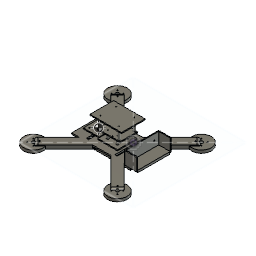
Drone Prototype Cad Model (Autodesk Fusion 360 design; units mm, degrees)
Autodesk Fusion 360 part; units mm, degrees
ref_plane "WorkPlane1" through (0, 0, 0) normal (0, 0, 1) x (1, 0, 0) in component "Standard_X_7in_Drone_OAKD_Pixhawk_Pi5_Final_Concept"
sketch "Arm_1_sketch" plane through (0, 0, 0) normal (0, 0, 1) x (1, 0, 0) in component "Standard_X_7in_Drone_OAKD_Pixhawk_Pi5_Final_Concept"
  line L0 (-10.6066, 10.6066) -> (121.9759, 143.1891)
  line L1 (121.9759, 143.1891) -> (143.1891, 121.9759)
  line L2 (143.1891, 121.9759) -> (10.6066, -10.6066)
  line L3 (10.6066, -10.6066) -> (-10.6066, 10.6066)
extrude "Extrude1" add sketch "Arm_1_sketch" along normal blind 12 makes body 1 in component "Standard_X_7in_Drone_OAKD_Pixhawk_Pi5_Final_Concept"
ref_plane "WorkPlane2" through (0, 0, 0) normal (0, 0, 1) x (1, 0, 0) in component "Standard_X_7in_Drone_OAKD_Pixhawk_Pi5_Final_Concept"
sketch "Arm_2_sketch" plane through (0, 0, 0) normal (0, 0, 1) x (1, 0, 0) in component "Standard_X_7in_Drone_OAKD_Pixhawk_Pi5_Final_Concept"
  line L0 (10.6066, 10.6066) -> (143.1891, -121.9759)
  line L1 (143.1891, -121.9759) -> (121.9759, -143.1891)
  line L2 (121.9759, -143.1891) -> (-10.6066, -10.6066)
  line L3 (-10.6066, -10.6066) -> (10.6066, 10.6066)
extrude "Extrude2" add sketch "Arm_2_sketch" along normal blind 12 separate body makes body 2 in component "Standard_X_7in_Drone_OAKD_Pixhawk_Pi5_Final_Concept"
ref_plane "WorkPlane3" through (0, 0, 0) normal (0, 0, 1) x (1, 0, 0) in component "Standard_X_7in_Drone_OAKD_Pixhawk_Pi5_Final_Concept"
sketch "Arm_3_sketch" plane through (0, 0, 0) normal (0, 0, 1) x (1, 0, 0) in component "Standard_X_7in_Drone_OAKD_Pixhawk_Pi5_Final_Concept"
  line L0 (10.6066, -10.6066) -> (-121.9759, -143.1891)
  line L1 (-121.9759, -143.1891) -> (-143.1891, -121.9759)
  line L2 (-143.1891, -121.9759) -> (-10.6066, 10.6066)
  line L3 (-10.6066, 10.6066) -> (10.6066, -10.6066)
extrude "Extrude3" add sketch "Arm_3_sketch" along normal blind 12 separate body makes body 3 in component "Standard_X_7in_Drone_OAKD_Pixhawk_Pi5_Final_Concept"
ref_plane "WorkPlane4" through (0, 0, 0) normal (0, 0, 1) x (1, 0, 0) in component "Standard_X_7in_Drone_OAKD_Pixhawk_Pi5_Final_Concept"
sketch "Arm_4_sketch" plane through (0, 0, 0) normal (0, 0, 1) x (1, 0, 0) in component "Standard_X_7in_Drone_OAKD_Pixhawk_Pi5_Final_Concept"
  line L0 (-10.6066, -10.6066) -> (-143.1891, 121.9759)
  line L1 (-143.1891, 121.9759) -> (-121.9759, 143.1891)
  line L2 (-121.9759, 143.1891) -> (10.6066, 10.6066)
  line L3 (10.6066, 10.6066) -> (-10.6066, -10.6066)
extrude "Extrude4" add sketch "Arm_4_sketch" along normal blind 12 separate body makes body 4 in component "Standard_X_7in_Drone_OAKD_Pixhawk_Pi5_Final_Concept"
ref_plane "WorkPlane5" through (0, 0, 0) normal (0, 0, 1) x (1, 0, 0) in component "Standard_X_7in_Drone_OAKD_Pixhawk_Pi5_Final_Concept"
sketch "Motor_Pad_1_sketch" plane through (0, 0, 0) normal (0, 0, 1) x (1, 0, 0) in component "Standard_X_7in_Drone_OAKD_Pixhawk_Pi5_Final_Concept"
  circle A0 centre (132.5825, 132.5825) radius 31
extrude "Extrude5" add sketch "Motor_Pad_1_sketch" along normal blind 9 separate body makes body 5 in component "Standard_X_7in_Drone_OAKD_Pixhawk_Pi5_Final_Concept"
ref_plane "WorkPlane6" through (0, 0, 0) normal (0, 0, 1) x (1, 0, 0) in component "Standard_X_7in_Drone_OAKD_Pixhawk_Pi5_Final_Concept"
sketch "Motor_Pad_2_sketch" plane through (0, 0, 0) normal (0, 0, 1) x (1, 0, 0) in component "Standard_X_7in_Drone_OAKD_Pixhawk_Pi5_Final_Concept"
  circle A0 centre (132.5825, -132.5825) radius 31
extrude "Extrude6" add sketch "Motor_Pad_2_sketch" along normal blind 9 separate body makes body 6 in component "Standard_X_7in_Drone_OAKD_Pixhawk_Pi5_Final_Concept"
ref_plane "WorkPlane7" through (0, 0, 0) normal (0, 0, 1) x (1, 0, 0) in component "Standard_X_7in_Drone_OAKD_Pixhawk_Pi5_Final_Concept"
sketch "Motor_Pad_3_sketch" plane through (0, 0, 0) normal (0, 0, 1) x (1, 0, 0) in component "Standard_X_7in_Drone_OAKD_Pixhawk_Pi5_Final_Concept"
  circle A0 centre (-132.5825, -132.5825) radius 31
extrude "Extrude7" add sketch "Motor_Pad_3_sketch" along normal blind 9 separate body makes body 7 in component "Standard_X_7in_Drone_OAKD_Pixhawk_Pi5_Final_Concept"
ref_plane "WorkPlane8" through (0, 0, 0) normal (0, 0, 1) x (1, 0, 0) in component "Standard_X_7in_Drone_OAKD_Pixhawk_Pi5_Final_Concept"
sketch "Motor_Pad_4_sketch" plane through (0, 0, 0) normal (0, 0, 1) x (1, 0, 0) in component "Standard_X_7in_Drone_OAKD_Pixhawk_Pi5_Final_Concept"
  circle A0 centre (-132.5825, 132.5825) radius 31
extrude "Extrude8" add sketch "Motor_Pad_4_sketch" along normal blind 9 separate body makes body 8 in component "Standard_X_7in_Drone_OAKD_Pixhawk_Pi5_Final_Concept"
ref_plane "WorkPlane9" through (0, 0, 8) normal (0, 0, 1) x (1, 0, 0) in component "Standard_X_7in_Drone_OAKD_Pixhawk_Pi5_Final_Concept"
sketch "Central_Lower_Body_Plate_sketch" plane through (0, 0, 8) normal (0, 0, 1) x (1, 0, 0) in component "Standard_X_7in_Drone_OAKD_Pixhawk_Pi5_Final_Concept"
  line L0 (-95, -50) -> (115, -50)
  line L1 (115, -50) -> (115, 50)
  line L2 (115, 50) -> (-95, 50)
  line L3 (-95, 50) -> (-95, -50)
  dimension "d213" = 95
  dimension "d214" = 50
  dimension "d215" = 210
  dimension "d216" = 100
  constraint perpendicular L0 L3
  constraint perpendicular L0 L1
  constraint perpendicular L1 L2
  constraint coincident L0.start L3.end
  constraint coincident L2.end L3.start
  constraint coincident L0.end L1.start
  constraint coincident L1.end L2.start
  constraint vertical L1
  measures "d213" distance of origin L3
  measures "d214" distance of origin L0
  measures "d215" distance of L1 L3
  measures "d216" distance of L0 L2
extrude "Extrude9" add sketch "Central_Lower_Body_Plate_sketch" along normal blind 4 separate body makes body 9 in component "Standard_X_7in_Drone_OAKD_Pixhawk_Pi5_Final_Concept"
ref_plane "WorkPlane10" through (0, 0, -18) normal (0, 0, 1) x (1, 0, 0) in component "Standard_X_7in_Drone_OAKD_Pixhawk_Pi5_Final_Concept"
sketch "Battery_Left_Rail_sketch" plane through (0, 0, -18) normal (0, 0, 1) x (1, 0, 0) in component "Standard_X_7in_Drone_OAKD_Pixhawk_Pi5_Final_Concept"
  line L0 (-83, -32) -> (67, -32)
  line L1 (67, -32) -> (67, -26)
  line L2 (67, -26) -> (-83, -26)
  line L3 (-83, -26) -> (-83, -32)
extrude "Extrude10" add sketch "Battery_Left_Rail_sketch" along normal blind 16 separate body makes body 10 in component "Standard_X_7in_Drone_OAKD_Pixhawk_Pi5_Final_Concept"
ref_plane "WorkPlane11" through (0, 0, -18) normal (0, 0, 1) x (1, 0, 0) in component "Standard_X_7in_Drone_OAKD_Pixhawk_Pi5_Final_Concept"
sketch "Battery_Right_Rail_sketch" plane through (0, 0, -18) normal (0, 0, 1) x (1, 0, 0) in component "Standard_X_7in_Drone_OAKD_Pixhawk_Pi5_Final_Concept"
  line L0 (-83, 26) -> (67, 26)
  line L1 (67, 26) -> (67, 32)
  line L2 (67, 32) -> (-83, 32)
  line L3 (-83, 32) -> (-83, 26)
extrude "Extrude11" add sketch "Battery_Right_Rail_sketch" along normal blind 16 separate body makes body 11 in component "Standard_X_7in_Drone_OAKD_Pixhawk_Pi5_Final_Concept"
ref_plane "WorkPlane12" through (0, 0, -18) normal (0, 0, 1) x (1, 0, 0) in component "Standard_X_7in_Drone_OAKD_Pixhawk_Pi5_Final_Concept"
sketch "Battery_Front_Stop_sketch" plane through (0, 0, -18) normal (0, 0, 1) x (1, 0, 0) in component "Standard_X_7in_Drone_OAKD_Pixhawk_Pi5_Final_Concept"
  line L0 (67, -32) -> (73, -32)
  line L1 (73, -32) -> (73, 32)
  line L2 (73, 32) -> (67, 32)
  line L3 (67, 32) -> (67, -32)
extrude "Extrude12" add sketch "Battery_Front_Stop_sketch" along normal blind 16 separate body makes body 12 in component "Standard_X_7in_Drone_OAKD_Pixhawk_Pi5_Final_Concept"
ref_plane "WorkPlane13" through (0, 0, -18) normal (0, 0, 1) x (1, 0, 0) in component "Standard_X_7in_Drone_OAKD_Pixhawk_Pi5_Final_Concept"
sketch "Battery_Rear_Stop_sketch" plane through (0, 0, -18) normal (0, 0, 1) x (1, 0, 0) in component "Standard_X_7in_Drone_OAKD_Pixhawk_Pi5_Final_Concept"
  line L0 (-89, -32) -> (-83, -32)
  line L1 (-83, -32) -> (-83, 32)
  line L2 (-83, 32) -> (-89, 32)
  line L3 (-89, 32) -> (-89, -32)
extrude "Extrude13" add sketch "Battery_Rear_Stop_sketch" along normal blind 16 separate body makes body 13 in component "Standard_X_7in_Drone_OAKD_Pixhawk_Pi5_Final_Concept"
ref_plane "WorkPlane14" through (0, 0, -58) normal (0, 0, 1) x (1, 0, 0) in component "Standard_X_7in_Drone_OAKD_Pixhawk_Pi5_Final_Concept"
sketch "Battery_Mockup_SOCOKIN_6S_4000mAh_Do_Not_Print_sketch" plane through (0, 0, -58) normal (0, 0, 1) x (1, 0, 0) in component "Standard_X_7in_Drone_OAKD_Pixhawk_Pi5_Final_Concept"
  line L0 (-78, -21.5) -> (62, -21.5)
  line L1 (62, -21.5) -> (62, 21.5)
  line L2 (62, 21.5) -> (-78, 21.5)
  line L3 (-78, 21.5) -> (-78, -21.5)
extrude "Extrude14" add sketch "Battery_Mockup_SOCOKIN_6S_4000mAh_Do_Not_Print_sketch" along normal blind 49 separate body makes body 14 in component "Standard_X_7in_Drone_OAKD_Pixhawk_Pi5_Final_Concept"
ref_plane "WorkPlane15" through (0, 0, 16) normal (0, 0, 1) x (1, 0, 0) in component "Standard_X_7in_Drone_OAKD_Pixhawk_Pi5_Final_Concept"
sketch "Tekko32_ESC_Lower_Mounting_Deck_sketch" plane through (0, 0, 16) normal (0, 0, 1) x (1, 0, 0) in component "Standard_X_7in_Drone_OAKD_Pixhawk_Pi5_Final_Concept"
  line L0 (-31, -31) -> (31, -31)
  line L1 (31, -31) -> (31, 31)
  line L2 (31, 31) -> (-31, 31)
  line L3 (-31, 31) -> (-31, -31)
extrude "Extrude15" add sketch "Tekko32_ESC_Lower_Mounting_Deck_sketch" along normal blind 3 separate body makes body 15 in component "Standard_X_7in_Drone_OAKD_Pixhawk_Pi5_Final_Concept"
ref_plane "WorkPlane16" through (0, 0, 19) normal (0, 0, 1) x (1, 0, 0) in component "Standard_X_7in_Drone_OAKD_Pixhawk_Pi5_Final_Concept"
sketch "Tekko32_ESC_Mockup_Do_Not_Print_sketch" plane through (0, 0, 19) normal (0, 0, 1) x (1, 0, 0) in component "Standard_X_7in_Drone_OAKD_Pixhawk_Pi5_Final_Concept"
  line L0 (-25, -25) -> (25, -25)
  line L1 (25, -25) -> (25, 25)
  line L2 (25, 25) -> (-25, 25)
  line L3 (-25, 25) -> (-25, -25)
extrude "Extrude16" add sketch "Tekko32_ESC_Mockup_Do_Not_Print_sketch" along normal blind 12 separate body makes body 16 in component "Standard_X_7in_Drone_OAKD_Pixhawk_Pi5_Final_Concept"
ref_plane "WorkPlane17" through (0, 0, 16) normal (0, 0, 1) x (1, 0, 0) in component "Standard_X_7in_Drone_OAKD_Pixhawk_Pi5_Final_Concept"
sketch "PM06_Power_Module_Mounting_Deck_sketch" plane through (0, 0, 16) normal (0, 0, 1) x (1, 0, 0) in component "Standard_X_7in_Drone_OAKD_Pixhawk_Pi5_Final_Concept"
  line L0 (-83, -25) -> (-33, -25)
  line L1 (-33, -25) -> (-33, 25)
  line L2 (-33, 25) -> (-83, 25)
  line L3 (-83, 25) -> (-83, -25)
extrude "Extrude17" add sketch "PM06_Power_Module_Mounting_Deck_sketch" along normal blind 3 separate body makes body 17 in component "Standard_X_7in_Drone_OAKD_Pixhawk_Pi5_Final_Concept"
ref_plane "WorkPlane18" through (0, 0, 19) normal (0, 0, 1) x (1, 0, 0) in component "Standard_X_7in_Drone_OAKD_Pixhawk_Pi5_Final_Concept"
sketch "PM06_Power_Module_Mockup_Do_Not_Print_sketch" plane through (0, 0, 19) normal (0, 0, 1) x (1, 0, 0) in component "Standard_X_7in_Drone_OAKD_Pixhawk_Pi5_Final_Concept"
  line L0 (-79, -21) -> (-37, -21)
  line L1 (-37, -21) -> (-37, 21)
  line L2 (-37, 21) -> (-79, 21)
  line L3 (-79, 21) -> (-79, -21)
extrude "Extrude18" add sketch "PM06_Power_Module_Mockup_Do_Not_Print_sketch" along normal blind 12 separate body makes body 18 in component "Standard_X_7in_Drone_OAKD_Pixhawk_Pi5_Final_Concept"
ref_plane "WorkPlane19" through (0, 0, 12) normal (0, 0, 1) x (1, 0, 0) in component "Standard_X_7in_Drone_OAKD_Pixhawk_Pi5_Final_Concept"
sketch "ESC_Deck_Standoff_1_sketch" plane through (0, 0, 12) normal (0, 0, 1) x (1, 0, 0) in component "Standard_X_7in_Drone_OAKD_Pixhawk_Pi5_Final_Concept"
  circle A0 centre (-15.25, -15.25) radius 3.5
extrude "Extrude19" add sketch "ESC_Deck_Standoff_1_sketch" along normal blind 4 separate body makes body 19 in component "Standard_X_7in_Drone_OAKD_Pixhawk_Pi5_Final_Concept"
ref_plane "WorkPlane20" through (0, 0, 12) normal (0, 0, 1) x (1, 0, 0) in component "Standard_X_7in_Drone_OAKD_Pixhawk_Pi5_Final_Concept"
sketch "ESC_Deck_Standoff_2_sketch" plane through (0, 0, 12) normal (0, 0, 1) x (1, 0, 0) in component "Standard_X_7in_Drone_OAKD_Pixhawk_Pi5_Final_Concept"
  circle A0 centre (15.25, -15.25) radius 3.5
extrude "Extrude20" add sketch "ESC_Deck_Standoff_2_sketch" along normal blind 4 separate body makes body 20 in component "Standard_X_7in_Drone_OAKD_Pixhawk_Pi5_Final_Concept"
ref_plane "WorkPlane21" through (0, 0, 12) normal (0, 0, 1) x (1, 0, 0) in component "Standard_X_7in_Drone_OAKD_Pixhawk_Pi5_Final_Concept"
sketch "ESC_Deck_Standoff_3_sketch" plane through (0, 0, 12) normal (0, 0, 1) x (1, 0, 0) in component "Standard_X_7in_Drone_OAKD_Pixhawk_Pi5_Final_Concept"
  circle A0 centre (-15.25, 15.25) radius 3.5
extrude "Extrude21" add sketch "ESC_Deck_Standoff_3_sketch" along normal blind 4 separate body makes body 21 in component "Standard_X_7in_Drone_OAKD_Pixhawk_Pi5_Final_Concept"
ref_plane "WorkPlane22" through (0, 0, 12) normal (0, 0, 1) x (1, 0, 0) in component "Standard_X_7in_Drone_OAKD_Pixhawk_Pi5_Final_Concept"
sketch "ESC_Deck_Standoff_4_sketch" plane through (0, 0, 12) normal (0, 0, 1) x (1, 0, 0) in component "Standard_X_7in_Drone_OAKD_Pixhawk_Pi5_Final_Concept"
  circle A0 centre (15.25, 15.25) radius 3.5
extrude "Extrude22" add sketch "ESC_Deck_Standoff_4_sketch" along normal blind 4 separate body makes body 22 in component "Standard_X_7in_Drone_OAKD_Pixhawk_Pi5_Final_Concept"
ref_plane "WorkPlane23" through (0, 0, 12) normal (0, 0, 1) x (1, 0, 0) in component "Standard_X_7in_Drone_OAKD_Pixhawk_Pi5_Final_Concept"
sketch "PM06_Deck_Standoff_1_sketch" plane through (0, 0, 12) normal (0, 0, 1) x (1, 0, 0) in component "Standard_X_7in_Drone_OAKD_Pixhawk_Pi5_Final_Concept"
  circle A0 centre (-73.25, -15.25) radius 3.5
extrude "Extrude23" add sketch "PM06_Deck_Standoff_1_sketch" along normal blind 4 separate body makes body 23 in component "Standard_X_7in_Drone_OAKD_Pixhawk_Pi5_Final_Concept"
ref_plane "WorkPlane24" through (0, 0, 12) normal (0, 0, 1) x (1, 0, 0) in component "Standard_X_7in_Drone_OAKD_Pixhawk_Pi5_Final_Concept"
sketch "PM06_Deck_Standoff_2_sketch" plane through (0, 0, 12) normal (0, 0, 1) x (1, 0, 0) in component "Standard_X_7in_Drone_OAKD_Pixhawk_Pi5_Final_Concept"
  circle A0 centre (-42.75, -15.25) radius 3.5
extrude "Extrude24" add sketch "PM06_Deck_Standoff_2_sketch" along normal blind 4 separate body makes body 24 in component "Standard_X_7in_Drone_OAKD_Pixhawk_Pi5_Final_Concept"
ref_plane "WorkPlane25" through (0, 0, 12) normal (0, 0, 1) x (1, 0, 0) in component "Standard_X_7in_Drone_OAKD_Pixhawk_Pi5_Final_Concept"
sketch "PM06_Deck_Standoff_3_sketch" plane through (0, 0, 12) normal (0, 0, 1) x (1, 0, 0) in component "Standard_X_7in_Drone_OAKD_Pixhawk_Pi5_Final_Concept"
  circle A0 centre (-73.25, 15.25) radius 3.5
extrude "Extrude25" add sketch "PM06_Deck_Standoff_3_sketch" along normal blind 4 separate body makes body 25 in component "Standard_X_7in_Drone_OAKD_Pixhawk_Pi5_Final_Concept"
ref_plane "WorkPlane26" through (0, 0, 12) normal (0, 0, 1) x (1, 0, 0) in component "Standard_X_7in_Drone_OAKD_Pixhawk_Pi5_Final_Concept"
sketch "PM06_Deck_Standoff_4_sketch" plane through (0, 0, 12) normal (0, 0, 1) x (1, 0, 0) in component "Standard_X_7in_Drone_OAKD_Pixhawk_Pi5_Final_Concept"
  circle A0 centre (-42.75, 15.25) radius 3.5
extrude "Extrude26" add sketch "PM06_Deck_Standoff_4_sketch" along normal blind 4 separate body makes body 26 in component "Standard_X_7in_Drone_OAKD_Pixhawk_Pi5_Final_Concept"
ref_plane "WorkPlane27" through (0, 0, 39) normal (0, 0, 1) x (1, 0, 0) in component "Standard_X_7in_Drone_OAKD_Pixhawk_Pi5_Final_Concept"
sketch "Pixhawk_6C_Mini_Isolated_Mounting_Deck_sketch" plane through (0, 0, 39) normal (0, 0, 1) x (1, 0, 0) in component "Standard_X_7in_Drone_OAKD_Pixhawk_Pi5_Final_Concept"
  line L0 (-36, -28) -> (36, -28)
  line L1 (36, -28) -> (36, 28)
  line L2 (36, 28) -> (-36, 28)
  line L3 (-36, 28) -> (-36, -28)
extrude "Extrude27" add sketch "Pixhawk_6C_Mini_Isolated_Mounting_Deck_sketch" along normal blind 3 separate body makes body 27 in component "Standard_X_7in_Drone_OAKD_Pixhawk_Pi5_Final_Concept"
ref_plane "WorkPlane28" through (0, 0, 42) normal (0, 0, 1) x (1, 0, 0) in component "Standard_X_7in_Drone_OAKD_Pixhawk_Pi5_Final_Concept"
sketch "Pixhawk_6C_Mini_Mockup_Do_Not_Print_sketch" plane through (0, 0, 42) normal (0, 0, 1) x (1, 0, 0) in component "Standard_X_7in_Drone_OAKD_Pixhawk_Pi5_Final_Concept"
  line L0 (-30, -22.5) -> (30, -22.5)
  line L1 (30, -22.5) -> (30, 22.5)
  line L2 (30, 22.5) -> (-30, 22.5)
  line L3 (-30, 22.5) -> (-30, -22.5)
extrude "Extrude28" add sketch "Pixhawk_6C_Mini_Mockup_Do_Not_Print_sketch" along normal blind 25 separate body makes body 28 in component "Standard_X_7in_Drone_OAKD_Pixhawk_Pi5_Final_Concept"
ref_plane "WorkPlane29" through (0, 0, 19) normal (0, 0, 1) x (1, 0, 0) in component "Standard_X_7in_Drone_OAKD_Pixhawk_Pi5_Final_Concept"
sketch "Pixhawk_Isolation_Standoff_1_sketch" plane through (0, 0, 19) normal (0, 0, 1) x (1, 0, 0) in component "Standard_X_7in_Drone_OAKD_Pixhawk_Pi5_Final_Concept"
  circle A0 centre (-15.25, -15.25) radius 3.5
extrude "Extrude29" add sketch "Pixhawk_Isolation_Standoff_1_sketch" along normal blind 20 separate body makes body 29 in component "Standard_X_7in_Drone_OAKD_Pixhawk_Pi5_Final_Concept"
ref_plane "WorkPlane30" through (0, 0, 19) normal (0, 0, 1) x (1, 0, 0) in component "Standard_X_7in_Drone_OAKD_Pixhawk_Pi5_Final_Concept"
sketch "Pixhawk_Isolation_Standoff_2_sketch" plane through (0, 0, 19) normal (0, 0, 1) x (1, 0, 0) in component "Standard_X_7in_Drone_OAKD_Pixhawk_Pi5_Final_Concept"
  circle A0 centre (15.25, -15.25) radius 3.5
extrude "Extrude30" add sketch "Pixhawk_Isolation_Standoff_2_sketch" along normal blind 20 separate body makes body 30 in component "Standard_X_7in_Drone_OAKD_Pixhawk_Pi5_Final_Concept"
ref_plane "WorkPlane31" through (0, 0, 19) normal (0, 0, 1) x (1, 0, 0) in component "Standard_X_7in_Drone_OAKD_Pixhawk_Pi5_Final_Concept"
sketch "Pixhawk_Isolation_Standoff_3_sketch" plane through (0, 0, 19) normal (0, 0, 1) x (1, 0, 0) in component "Standard_X_7in_Drone_OAKD_Pixhawk_Pi5_Final_Concept"
  circle A0 centre (-15.25, 15.25) radius 3.5
extrude "Extrude31" add sketch "Pixhawk_Isolation_Standoff_3_sketch" along normal blind 20 separate body makes body 31 in component "Standard_X_7in_Drone_OAKD_Pixhawk_Pi5_Final_Concept"
ref_plane "WorkPlane32" through (0, 0, 19) normal (0, 0, 1) x (1, 0, 0) in component "Standard_X_7in_Drone_OAKD_Pixhawk_Pi5_Final_Concept"
sketch "Pixhawk_Isolation_Standoff_4_sketch" plane through (0, 0, 19) normal (0, 0, 1) x (1, 0, 0) in component "Standard_X_7in_Drone_OAKD_Pixhawk_Pi5_Final_Concept"
  circle A0 centre (15.25, 15.25) radius 3.5
extrude "Extrude32" add sketch "Pixhawk_Isolation_Standoff_4_sketch" along normal blind 20 separate body makes body 32 in component "Standard_X_7in_Drone_OAKD_Pixhawk_Pi5_Final_Concept"
ref_plane "WorkPlane33" through (0, 0, 76) normal (0, 0, 1) x (1, 0, 0) in component "Standard_X_7in_Drone_OAKD_Pixhawk_Pi5_Final_Concept"
sketch "Raspberry_Pi_5_Upper_Deck_sketch" plane through (0, 0, 76) normal (0, 0, 1) x (1, 0, 0) in component "Standard_X_7in_Drone_OAKD_Pixhawk_Pi5_Final_Concept"
  line L0 (-70, -37.5) -> (30, -37.5)
  line L1 (30, -37.5) -> (30, 37.5)
  line L2 (30, 37.5) -> (-70, 37.5)
  line L3 (-70, 37.5) -> (-70, -37.5)
extrude "Extrude33" add sketch "Raspberry_Pi_5_Upper_Deck_sketch" along normal blind 3 separate body makes body 33 in component "Standard_X_7in_Drone_OAKD_Pixhawk_Pi5_Final_Concept"
ref_plane "WorkPlane34" through (0, 0, 79) normal (0, 0, 1) x (1, 0, 0) in component "Standard_X_7in_Drone_OAKD_Pixhawk_Pi5_Final_Concept"
sketch "Raspberry_Pi_5_Mockup_With_Cooler_Clearance_Do_Not_Print_sketch" plane through (0, 0, 79) normal (0, 0, 1) x (1, 0, 0) in component "Standard_X_7in_Drone_OAKD_Pixhawk_Pi5_Final_Concept"
  line L0 (-65, -32.5) -> (25, -32.5)
  line L1 (25, -32.5) -> (25, 32.5)
  line L2 (25, 32.5) -> (-65, 32.5)
  line L3 (-65, 32.5) -> (-65, -32.5)
extrude "Extrude34" add sketch "Raspberry_Pi_5_Mockup_With_Cooler_Clearance_Do_Not_Print_sketch" along normal blind 25 separate body makes body 34 in component "Standard_X_7in_Drone_OAKD_Pixhawk_Pi5_Final_Concept"
ref_plane "WorkPlane35" through (0, 0, 42) normal (0, 0, 1) x (1, 0, 0) in component "Standard_X_7in_Drone_OAKD_Pixhawk_Pi5_Final_Concept"
sketch "Pi_Upper_Deck_Standoff_1_sketch" plane through (0, 0, 42) normal (0, 0, 1) x (1, 0, 0) in component "Standard_X_7in_Drone_OAKD_Pixhawk_Pi5_Final_Concept"
  circle A0 centre (-49, -24.5) radius 3.5
extrude "Extrude35" add sketch "Pi_Upper_Deck_Standoff_1_sketch" along normal blind 34 separate body makes body 35 in component "Standard_X_7in_Drone_OAKD_Pixhawk_Pi5_Final_Concept"
ref_plane "WorkPlane36" through (0, 0, 42) normal (0, 0, 1) x (1, 0, 0) in component "Standard_X_7in_Drone_OAKD_Pixhawk_Pi5_Final_Concept"
sketch "Pi_Upper_Deck_Standoff_2_sketch" plane through (0, 0, 42) normal (0, 0, 1) x (1, 0, 0) in component "Standard_X_7in_Drone_OAKD_Pixhawk_Pi5_Final_Concept"
  circle A0 centre (9, -24.5) radius 3.5
extrude "Extrude36" add sketch "Pi_Upper_Deck_Standoff_2_sketch" along normal blind 34 separate body makes body 36 in component "Standard_X_7in_Drone_OAKD_Pixhawk_Pi5_Final_Concept"
ref_plane "WorkPlane37" through (0, 0, 42) normal (0, 0, 1) x (1, 0, 0) in component "Standard_X_7in_Drone_OAKD_Pixhawk_Pi5_Final_Concept"
sketch "Pi_Upper_Deck_Standoff_3_sketch" plane through (0, 0, 42) normal (0, 0, 1) x (1, 0, 0) in component "Standard_X_7in_Drone_OAKD_Pixhawk_Pi5_Final_Concept"
  circle A0 centre (-49, 24.5) radius 3.5
extrude "Extrude37" add sketch "Pi_Upper_Deck_Standoff_3_sketch" along normal blind 34 separate body makes body 37 in component "Standard_X_7in_Drone_OAKD_Pixhawk_Pi5_Final_Concept"
ref_plane "WorkPlane38" through (0, 0, 42) normal (0, 0, 1) x (1, 0, 0) in component "Standard_X_7in_Drone_OAKD_Pixhawk_Pi5_Final_Concept"
sketch "Pi_Upper_Deck_Standoff_4_sketch" plane through (0, 0, 42) normal (0, 0, 1) x (1, 0, 0) in component "Standard_X_7in_Drone_OAKD_Pixhawk_Pi5_Final_Concept"
  circle A0 centre (9, 24.5) radius 3.5
extrude "Extrude38" add sketch "Pi_Upper_Deck_Standoff_4_sketch" along normal blind 34 separate body makes body 38 in component "Standard_X_7in_Drone_OAKD_Pixhawk_Pi5_Final_Concept"
ref_plane "WorkPlane39" through (0, 0, 39) normal (0, 0, 1) x (1, 0, 0) in component "Standard_X_7in_Drone_OAKD_Pixhawk_Pi5_Final_Concept"
sketch "Separate_5V_BEC_Mounting_Platform_sketch" plane through (0, 0, 39) normal (0, 0, 1) x (1, 0, 0) in component "Standard_X_7in_Drone_OAKD_Pixhawk_Pi5_Final_Concept"
  line L0 (33, 21) -> (75, 21)
  line L1 (75, 21) -> (75, 47)
  line L2 (75, 47) -> (33, 47)
  line L3 (33, 47) -> (33, 21)
extrude "Extrude39" add sketch "Separate_5V_BEC_Mounting_Platform_sketch" along normal blind 3 separate body makes body 39 in component "Standard_X_7in_Drone_OAKD_Pixhawk_Pi5_Final_Concept"
ref_plane "WorkPlane40" through (0, 0, 42) normal (0, 0, 1) x (1, 0, 0) in component "Standard_X_7in_Drone_OAKD_Pixhawk_Pi5_Final_Concept"
sketch "5V_BEC_Mockup_For_Pi5_And_OAKD_Do_Not_Print_sketch" plane through (0, 0, 42) normal (0, 0, 1) x (1, 0, 0) in component "Standard_X_7in_Drone_OAKD_Pixhawk_Pi5_Final_Concept"
  line L0 (36, 24) -> (72, 24)
  line L1 (72, 24) -> (72, 44)
  line L2 (72, 44) -> (36, 44)
  line L3 (36, 44) -> (36, 24)
extrude "Extrude40" add sketch "5V_BEC_Mockup_For_Pi5_And_OAKD_Do_Not_Print_sketch" along normal blind 10 separate body makes body 40 in component "Standard_X_7in_Drone_OAKD_Pixhawk_Pi5_Final_Concept"
ref_plane "WorkPlane41" through (0, 0, 39) normal (0, 0, 1) x (1, 0, 0) in component "Standard_X_7in_Drone_OAKD_Pixhawk_Pi5_Final_Concept"
sketch "RadioMaster_RP1_Receiver_Platform_sketch" plane through (0, 0, 39) normal (0, 0, 1) x (1, 0, 0) in component "Standard_X_7in_Drone_OAKD_Pixhawk_Pi5_Final_Concept"
  line L0 (-100, 22) -> (-68, 22)
  line L1 (-68, 22) -> (-68, 46)
  line L2 (-68, 46) -> (-100, 46)
  line L3 (-100, 46) -> (-100, 22)
ref_plane "WorkPlane42" through (0, 0, 41.5) normal (0, 0, 1) x (1, 0, 0) in component "Standard_X_7in_Drone_OAKD_Pixhawk_Pi5_Final_Concept"
sketch "RadioMaster_RP1_Receiver_Mockup_Do_Not_Print_sketch" plane through (0, 0, 41.5) normal (0, 0, 1) x (1, 0, 0) in component "Standard_X_7in_Drone_OAKD_Pixhawk_Pi5_Final_Concept"
  line L0 (-96.5, 24) -> (-71.5, 24)
  line L1 (-71.5, 24) -> (-71.5, 44)
  line L2 (-71.5, 44) -> (-96.5, 44)
  line L3 (-96.5, 44) -> (-96.5, 24)
ref_plane "WorkPlane43" through (0, 0, 39) normal (0, 0, 1) x (1, 0, 0) in component "Standard_X_7in_Drone_OAKD_Pixhawk_Pi5_Final_Concept"
sketch "RP1_Antenna_Guide_Post_sketch" plane through (0, 0, 39) normal (0, 0, 1) x (1, 0, 0) in component "Standard_X_7in_Drone_OAKD_Pixhawk_Pi5_Final_Concept"
  circle A0 centre (-94, 46) radius 1.5
ref_plane "WorkPlane44" through (0, 0, 24) normal (0, 0, 1) x (1, 0, 0) in component "Standard_X_7in_Drone_OAKD_Pixhawk_Pi5_Final_Concept"
sketch "OAKD_Lite_Front_Camera_Bottom_Shelf_sketch" plane through (0, 0, 24) normal (0, 0, 1) x (1, 0, 0) in component "Standard_X_7in_Drone_OAKD_Pixhawk_Pi5_Final_Concept"
  line L0 (100, -53) -> (138, -53)
  line L1 (138, -53) -> (138, 53)
  line L2 (138, 53) -> (100, 53)
  line L3 (100, 53) -> (100, -53)
extrude "Extrude44" add sketch "OAKD_Lite_Front_Camera_Bottom_Shelf_sketch" along normal blind 3 separate body makes body 41 in component "Standard_X_7in_Drone_OAKD_Pixhawk_Pi5_Final_Concept"
ref_plane "WorkPlane45" through (0, 0, 24) normal (0, 0, 1) x (1, 0, 0) in component "Standard_X_7in_Drone_OAKD_Pixhawk_Pi5_Final_Concept"
sketch "OAKD_Lite_Front_Camera_Left_Cheek_sketch" plane through (0, 0, 24) normal (0, 0, 1) x (1, 0, 0) in component "Standard_X_7in_Drone_OAKD_Pixhawk_Pi5_Final_Concept"
  line L0 (100, -54.5) -> (138, -54.5)
  line L1 (138, -54.5) -> (138, -51.5)
  line L2 (138, -51.5) -> (100, -51.5)
  line L3 (100, -51.5) -> (100, -54.5)
extrude "Extrude45" add sketch "OAKD_Lite_Front_Camera_Left_Cheek_sketch" along normal blind 40 separate body makes body 42 in component "Standard_X_7in_Drone_OAKD_Pixhawk_Pi5_Final_Concept"
ref_plane "WorkPlane46" through (0, 0, 24) normal (0, 0, 1) x (1, 0, 0) in component "Standard_X_7in_Drone_OAKD_Pixhawk_Pi5_Final_Concept"
sketch "OAKD_Lite_Front_Camera_Right_Cheek_sketch" plane through (0, 0, 24) normal (0, 0, 1) x (1, 0, 0) in component "Standard_X_7in_Drone_OAKD_Pixhawk_Pi5_Final_Concept"
  line L0 (100, 51.5) -> (138, 51.5)
  line L1 (138, 51.5) -> (138, 54.5)
  line L2 (138, 54.5) -> (100, 54.5)
  line L3 (100, 54.5) -> (100, 51.5)
extrude "Extrude46" add sketch "OAKD_Lite_Front_Camera_Right_Cheek_sketch" along normal blind 40 separate body makes body 43 in component "Standard_X_7in_Drone_OAKD_Pixhawk_Pi5_Final_Concept"
ref_plane "WorkPlane47" through (0, 0, 24) normal (0, 0, 1) x (1, 0, 0) in component "Standard_X_7in_Drone_OAKD_Pixhawk_Pi5_Final_Concept"
sketch "OAKD_Lite_Camera_Rear_Brace_sketch" plane through (0, 0, 24) normal (0, 0, 1) x (1, 0, 0) in component "Standard_X_7in_Drone_OAKD_Pixhawk_Pi5_Final_Concept"
  line L0 (98.5, -53) -> (101.5, -53)
  line L1 (101.5, -53) -> (101.5, 53)
  line L2 (101.5, 53) -> (98.5, 53)
  line L3 (98.5, 53) -> (98.5, -53)
extrude "Extrude47" add sketch "OAKD_Lite_Camera_Rear_Brace_sketch" along normal blind 40 separate body makes body 44 in component "Standard_X_7in_Drone_OAKD_Pixhawk_Pi5_Final_Concept"
ref_plane "WorkPlane48" through (0, 0, 28) normal (0, 0, 1) x (1, 0, 0) in component "Standard_X_7in_Drone_OAKD_Pixhawk_Pi5_Final_Concept"
sketch "OAKD_Lite_Clearance_Mockup_Do_Not_Print_sketch" plane through (0, 0, 28) normal (0, 0, 1) x (1, 0, 0) in component "Standard_X_7in_Drone_OAKD_Pixhawk_Pi5_Final_Concept"
  line L0 (107, -48) -> (135, -48)
  line L1 (135, -48) -> (135, 48)
  line L2 (135, 48) -> (107, 48)
  line L3 (107, 48) -> (107, -48)
extrude "Extrude48" add sketch "OAKD_Lite_Clearance_Mockup_Do_Not_Print_sketch" along normal blind 34 separate body makes body 45 in component "Standard_X_7in_Drone_OAKD_Pixhawk_Pi5_Final_Concept"
ref_plane "WorkPlane49" through (0, 0, -1) normal (0, 0, 1) x (1, 0, 0) in component "Standard_X_7in_Drone_OAKD_Pixhawk_Pi5_Final_Concept"
sketch "Motor_Mount_Hole_Cut_Sketch" plane through (0, 0, -1) normal (0, 0, 1) x (1, 0, 0) in component "Standard_X_7in_Drone_OAKD_Pixhawk_Pi5_Final_Concept"
  circle A0 centre (132.5825, 132.5825) radius 5
  circle A1 centre (123.0825, 123.0825) radius 1.7
  circle A2 centre (142.0825, 123.0825) radius 1.7
  circle A3 centre (123.0825, 142.0825) radius 1.7
  circle A4 centre (142.0825, 142.0825) radius 1.7
  circle A5 centre (132.5825, -132.5825) radius 5
  circle A6 centre (123.0825, -142.0825) radius 1.7
  circle A7 centre (142.0825, -142.0825) radius 1.7
  circle A8 centre (123.0825, -123.0825) radius 1.7
  circle A9 centre (142.0825, -123.0825) radius 1.7
  circle A10 centre (-132.5825, -132.5825) radius 5
  circle A11 centre (-142.0825, -142.0825) radius 1.7
  circle A12 centre (-123.0825, -142.0825) radius 1.7
  circle A13 centre (-142.0825, -123.0825) radius 1.7
  circle A14 centre (-123.0825, -123.0825) radius 1.7
  circle A15 centre (-132.5825, 132.5825) radius 5
  circle A16 centre (-142.0825, 123.0825) radius 1.7
  circle A17 centre (-123.0825, 123.0825) radius 1.7
  circle A18 centre (-142.0825, 142.0825) radius 1.7
  circle A19 centre (-123.0825, 142.0825) radius 1.7
extrude "Extrude49" cut sketch "Motor_Mount_Hole_Cut_Sketch" along normal blind 12 bodies 1 2 3 4 5 6 7 8 in component "Standard_X_7in_Drone_OAKD_Pixhawk_Pi5_Final_Concept"
ref_plane "WorkPlane50" through (0, 0, 7) normal (0, 0, 1) x (1, 0, 0) in component "Standard_X_7in_Drone_OAKD_Pixhawk_Pi5_Final_Concept"
sketch "Battery_Strap_Slot_Cut_Sketch" plane through (0, 0, 7) normal (0, 0, 1) x (1, 0, 0) in component "Standard_X_7in_Drone_OAKD_Pixhawk_Pi5_Final_Concept"
  line L0 (-56.5, -41) -> (-49.5, -41)
  line L1 (-49.5, -41) -> (-49.5, 41)
  line L2 (-49.5, 41) -> (-56.5, 41)
  line L3 (-56.5, 41) -> (-56.5, -41)
  line L4 (33.5, -41) -> (40.5, -41)
  line L5 (40.5, -41) -> (40.5, 41)
  line L6 (40.5, 41) -> (33.5, 41)
  line L7 (33.5, 41) -> (33.5, -41)
extrude "Extrude50" cut sketch "Battery_Strap_Slot_Cut_Sketch" along normal blind 8 bodies 1 2 3 4 9 in component "Standard_X_7in_Drone_OAKD_Pixhawk_Pi5_Final_Concept"
ref_plane "WorkPlane51" through (0, 0, 11) normal (0, 0, 1) x (1, 0, 0) in component "Standard_X_7in_Drone_OAKD_Pixhawk_Pi5_Final_Concept"
sketch "Electronics_Stack_Hole_Cut_Sketch" plane through (0, 0, 11) normal (0, 0, 1) x (1, 0, 0) in component "Standard_X_7in_Drone_OAKD_Pixhawk_Pi5_Final_Concept"
  circle A0 centre (-15.25, -15.25) radius 1.6
  circle A1 centre (15.25, -15.25) radius 1.6
  circle A2 centre (-15.25, 15.25) radius 1.6
  circle A3 centre (15.25, 15.25) radius 1.6
  circle A4 centre (-73.25, -15.25) radius 1.6
  circle A5 centre (-42.75, -15.25) radius 1.6
  circle A6 centre (-73.25, 15.25) radius 1.6
  circle A7 centre (-42.75, 15.25) radius 1.6
  circle A8 centre (-15.25, -15.25) radius 1.6
  circle A9 centre (15.25, -15.25) radius 1.6
  circle A10 centre (-15.25, 15.25) radius 1.6
  circle A11 centre (15.25, 15.25) radius 1.6
extrude "Extrude51" cut sketch "Electronics_Stack_Hole_Cut_Sketch" along normal blind 47 bodies 1 2 3 4 9 15 16 17 18 19 20 21 22 23 24 25 26 27 28 29 30 31 32 in component "Standard_X_7in_Drone_OAKD_Pixhawk_Pi5_Final_Concept"
ref_plane "WorkPlane52" through (0, 0, 41) normal (0, 0, 1) x (1, 0, 0) in component "Standard_X_7in_Drone_OAKD_Pixhawk_Pi5_Final_Concept"
sketch "Raspberry_Pi_5_Mounting_Hole_Cut_Sketch" plane through (0, 0, 41) normal (0, 0, 1) x (1, 0, 0) in component "Standard_X_7in_Drone_OAKD_Pixhawk_Pi5_Final_Concept"
  circle A0 centre (-49, -24.5) radius 1.4
  circle A1 centre (9, -24.5) radius 1.4
  circle A2 centre (-49, 24.5) radius 1.4
  circle A3 centre (9, 24.5) radius 1.4
extrude "Extrude52" cut sketch "Raspberry_Pi_5_Mounting_Hole_Cut_Sketch" along normal blind 84 bodies 27 33 34 35 36 37 38 in component "Standard_X_7in_Drone_OAKD_Pixhawk_Pi5_Final_Concept"
sketch "7in_Propeller_Clearance_Circles_Do_Not_Print" plane through (0, 0, 0) normal (0, 0, 1) x (1, 0, 0) in component "Standard_X_7in_Drone_OAKD_Pixhawk_Pi5_Final_Concept"
  circle A0 centre (132.5825, 132.5825) radius 88.9
  circle A1 centre (132.5825, -132.5825) radius 88.9
  circle A2 centre (-132.5825, -132.5825) radius 88.9
  circle A3 centre (-132.5825, 132.5825) radius 88.9
sketch "OAKD_Lite_Horizontal_FOV_Guide_Do_Not_Print" plane through (0, 0, 0) normal (0, 0, 1) x (1, 0, 0) in component "Standard_X_7in_Drone_OAKD_Pixhawk_Pi5_Final_Concept"
  line L0 (133, 0) -> (353, 0)
  line L1 (133, 0) -> (309.8485, 130.861)
  line L2 (133, 0) -> (309.8485, -130.861)
ref_plane "WorkPlane53" through (0, 0, -3) normal (0, 0, 1) x (1, 0, 0) in component "Standard_X_7in_Drone_OAKD_Pixhawk_Pi5_Final_Concept"
sketch "Center_Reference_Marker_Do_Not_Print_sketch" plane through (0, 0, -3) normal (0, 0, 1) x (1, 0, 0) in component "Standard_X_7in_Drone_OAKD_Pixhawk_Pi5_Final_Concept"
  circle A0 centre (0, 0) radius 4
extrude "Extrude53" add sketch "Center_Reference_Marker_Do_Not_Print_sketch" along normal blind 2 separate body makes body 46 in component "Standard_X_7in_Drone_OAKD_Pixhawk_Pi5_Final_Concept"
move_body "Move1" bodies 44 43 42 41 to x (1, 0, 0) y (0, 1, 0) z (0, 0, 1) at (-18, 0, 0) in component "Standard_X_7in_Drone_OAKD_Pixhawk_Pi5_Final_Concept"
combine "Combine1" operation add target body 1 tool bodies 9 4 3 2 in component "Standard_X_7in_Drone_OAKD_Pixhawk_Pi5_Final_Concept"
move_body "Move2" bodies 42 41 43 44 to x (1, 0, 0) y (0, 1, 0) z (0, 0, 1) at (0, 0, -10) in component "Standard_X_7in_Drone_OAKD_Pixhawk_Pi5_Final_Concept"
move_body "Move3" bodies 42 41 43 44 to x (1, 0, 0) y (0, 1, 0) z (0, 0, 1) at (-5, 0, -2) in component "Standard_X_7in_Drone_OAKD_Pixhawk_Pi5_Final_Concept"
combine "Combine2" operation add target body 42 tool bodies 41 44 1 in component "Standard_X_7in_Drone_OAKD_Pixhawk_Pi5_Final_Concept"
fillet "Fillet1" radius 5 4 edges at (27.3566, 6.1434, 8) (27.3566, -6.1434, 8) (-35.3566, 14.1434, 8) (-35.3566, -14.1434, 8) on bodies 42 in component "Standard_X_7in_Drone_OAKD_Pixhawk_Pi5_Final_Concept"
fillet "Fillet2" radius 5 4 edges at (-14.3934, 35.6066, 8) (14.3934, 35.6066, 8) (14.3934, -35.6066, 8) (-14.3934, -35.6066, 8) on bodies 42 in component "Standard_X_7in_Drone_OAKD_Pixhawk_Pi5_Final_Concept"
hole "Hole3" at (78.5, -37.5, 33.5) direction (-1, 0, 0) diameter 4 depth 20 tip angle 180 bodies 42 in component "Standard_X_7in_Drone_OAKD_Pixhawk_Pi5_Final_Concept"
hole "Hole4" at (78.5, 37.5, 33.5) direction (-1, 0, 0) diameter 4 depth 20 tip angle 180 bodies 42 in component "Standard_X_7in_Drone_OAKD_Pixhawk_Pi5_Final_Concept"
combine "Combine3" operation add target body 11 tool bodies 12 10 13 in component "Standard_X_7in_Drone_OAKD_Pixhawk_Pi5_Final_Concept"
move_body "Move4" bodies 11 to x (1, 0, 0) y (0, 1, 0) z (0, 0, 1) at (0, 0, 2) in component "Standard_X_7in_Drone_OAKD_Pixhawk_Pi5_Final_Concept"
move_body "Move5" bodies 39 to x (0, 1, 0) y (-1, 0, 0) z (0, 0, 1) at (91.7542, -26.4756, 0) in component "Standard_X_7in_Drone_OAKD_Pixhawk_Pi5_Final_Concept"
move_body "Move6" bodies 39 to x (1, 0, 0) y (0, 1, 0) z (0, 0, 1) at (0, 0, -27) in component "Standard_X_7in_Drone_OAKD_Pixhawk_Pi5_Final_Concept"
combine "Combine4" operation add target body 33 tool bodies 37 38 35 36 in component "Standard_X_7in_Drone_OAKD_Pixhawk_Pi5_Final_Concept"
hole "Hole5" at (123.1532, 122.9914, 11) direction (0, 0, 1) diameter 3 depth 1.7 tip angle 118 bodies 42 in component "Standard_X_7in_Drone_OAKD_Pixhawk_Pi5_Final_Concept"
hole "Hole8" at (-122.977, 123.2327, 11) direction (0, 0, 1) diameter 3 depth 1.7 tip angle 118 bodies 42 in component "Standard_X_7in_Drone_OAKD_Pixhawk_Pi5_Final_Concept"
hole "Hole9" at (122.6888, -122.0287, 11) direction (0, 0, 1) diameter 3 depth 1.7 tip angle 118 bodies 42 in component "Standard_X_7in_Drone_OAKD_Pixhawk_Pi5_Final_Concept"
hole "Hole10" at (-123.4213, -122.2526, 11) direction (0, 0, 1) diameter 3 depth 1.7 tip angle 118 bodies 42 in component "Standard_X_7in_Drone_OAKD_Pixhawk_Pi5_Final_Concept"
fillet "Fillet3" radius 10 1 edges at (132.5825, 132.5825, 12) on bodies 42 in component "Standard_X_7in_Drone_OAKD_Pixhawk_Pi5_Final_Concept"
fillet "Fillet4" radius 10 1 edges at (-132.5825, 132.5825, 12) on bodies 42 in component "Standard_X_7in_Drone_OAKD_Pixhawk_Pi5_Final_Concept"
fillet "Fillet5" radius 10 1 edges at (-132.5825, -132.5825, 12) on bodies 42 in component "Standard_X_7in_Drone_OAKD_Pixhawk_Pi5_Final_Concept"
fillet "Fillet6" radius 10 1 edges at (132.5825, -132.5825, 12) on bodies 42 in component "Standard_X_7in_Drone_OAKD_Pixhawk_Pi5_Final_Concept"
combine "Combine5" [suppressed] in component "Standard_X_7in_Drone_OAKD_Pixhawk_Pi5_Final_Concept"
combine "Combine6" [suppressed] in component "Standard_X_7in_Drone_OAKD_Pixhawk_Pi5_Final_Concept"
combine "Combine7" [suppressed] in component "Standard_X_7in_Drone_OAKD_Pixhawk_Pi5_Final_Concept"
combine "Combine8" [suppressed] in component "Standard_X_7in_Drone_OAKD_Pixhawk_Pi5_Final_Concept"
combine "Combine9" [suppressed] in component "Standard_X_7in_Drone_OAKD_Pixhawk_Pi5_Final_Concept"
combine "Combine10" [suppressed] in component "Standard_X_7in_Drone_OAKD_Pixhawk_Pi5_Final_Concept"
combine "Combine11" [suppressed] in component "Standard_X_7in_Drone_OAKD_Pixhawk_Pi5_Final_Concept"
move_body "Move8" bodies 33 42 43 25 26 17 5 6 11 22 7 24 23 15 32 27 30 29 31 21 20 19 8 to x (1, 0, 0) y (0, 0, -1) z (0, 1, 0) at (0, 12, 50) in component "Standard_X_7in_Drone_OAKD_Pixhawk_Pi5_Final_Concept"
move_body "Move9" bodies 17 43 5 22 26 25 24 23 15 32 27 30 29 31 21 20 19 8 7 6 11 33 42 to x (1, 0, 0) y (0, 1, 0) z (0, 0, 1) at (0, 5, 0) in component "Standard_X_7in_Drone_OAKD_Pixhawk_Pi5_Final_Concept"
combine "Combine12" operation add target body 42 tool bodies 43 5 8 7 6 11 in component "Standard_X_7in_Drone_OAKD_Pixhawk_Pi5_Final_Concept"
move_body "Move10" bodies 33 to x (1, 0, 0) y (0, 1, 0) z (0, 0, 1) at (20, 0, 0) in component "Standard_X_7in_Drone_OAKD_Pixhawk_Pi5_Final_Concept"
hole "Hole14" at (-29.17, 59, 74.589) direction (0, -1, 0) diameter 2.5 depth 15 tip angle 180 bodies 27 in component "Standard_X_7in_Drone_OAKD_Pixhawk_Pi5_Final_Concept"
hole "Hole15" at (-29.17, 59, 25.411) direction (0, -1, 0) diameter 2.5 depth 15 tip angle 180 bodies 27 in component "Standard_X_7in_Drone_OAKD_Pixhawk_Pi5_Final_Concept"
hole "Hole16" at (29.17, 59, 25.4111) direction (0, -1, 0) diameter 2.5 depth 15 tip angle 180 bodies 27 in component "Standard_X_7in_Drone_OAKD_Pixhawk_Pi5_Final_Concept"
move_body "Move11" bodies 33 to x (1, 0, 0) y (0, 1, 0) z (0, 0, 1) at (30, 0, 0) in component "Standard_X_7in_Drone_OAKD_Pixhawk_Pi5_Final_Concept"
move_body "Move12" bodies 33 to x (1, 0, 0) y (0, 1, 0) z (0, 0, 1) at (-29.83, 0, -0.0889) in component "Standard_X_7in_Drone_OAKD_Pixhawk_Pi5_Final_Concept"
hole "Hole17" at (29.17, 59, 74.589) direction (0, -1, 0) diameter 2.6 depth 15 tip angle 180 bodies 27 in component "Standard_X_7in_Drone_OAKD_Pixhawk_Pi5_Final_Concept"
sketch "Sketch2" plane through (0, 0, 0) normal (0, 1, 0) x (1, 0, 0)
  line L0 (180, 180) -> (-180, 180)
  line L1 (-180, 180) -> (-180, -180)
  line L2 (-180, -180) -> (180, -180)
  line L3 (180, -180) -> (180, 180)
  line L4 (180, 180) -> (-180, -180) construction
  line L5 (-180, 180) -> (180, -180) construction
  dimension "d298" = 360
  dimension "d299" = 360
  constraint horizontal L0
  constraint perpendicular L0 L1
  constraint parallel L0 L2
  constraint parallel L1 L3
  constraint coincident L4 origin
  constraint coincident L5 origin
  measures "d298" distance of L0.start L0.end
  measures "d299" distance of L0.end L1.end
combine "Combine14" operation add target body 27 tool bodies 29 31 30 32 in component "Standard_X_7in_Drone_OAKD_Pixhawk_Pi5_Final_Concept"
combine "Combine15" operation add target body 15 tool bodies 22 21 19 20 in component "Standard_X_7in_Drone_OAKD_Pixhawk_Pi5_Final_Concept"
component "Standard_X_7in_Drone_OAKD_Pixhawk_Pi5_Final_Concept" placed x (1, 0, 0) y (0, 1, 0) z (0, 0, 1) at (0, 0, 0)
hidden bodies 14 16 18 28 34 39 40 45 46
named bodies: "Arm_1", "Arm_2", "Arm_3", "Arm_4", "Motor_Pad_1", "Motor_Pad_2", "Motor_Pad_3", "Motor_Pad_4", "Central_Lower_Body_Plate", "Battery_Left_Rail", "Battery_Right_Rail", "Battery_Front_Stop", "Battery_Rear_Stop", "Battery_Mockup_SOCOKIN_6S_4000mAh_Do_Not_Print", "Tekko32_ESC_Lower_Mounting_Deck", "Tekko32_ESC_Mockup_Do_Not_Print", "PM06_Power_Module_Mounting_Deck", "PM06_Power_Module_Mockup_Do_Not_Print", "ESC_Deck_Standoff_1", "ESC_Deck_Standoff_2", "ESC_Deck_Standoff_3", "ESC_Deck_Standoff_4", "PM06_Deck_Standoff_1", "PM06_Deck_Standoff_2", "PM06_Deck_Standoff_3", "PM06_Deck_Standoff_4", "Pixhawk_6C_Mini_Isolated_Mounting_Deck", "Pixhawk_6C_Mini_Mockup_Do_Not_Print", "Pixhawk_Isolation_Standoff_1", "Pixhawk_Isolation_Standoff_2", "Pixhawk_Isolation_Standoff_3", "Pixhawk_Isolation_Standoff_4", "Raspberry_Pi_5_Upper_Deck", "Raspberry_Pi_5_Mockup_With_Cooler_Clearance_Do_Not_Print", "Pi_Upper_Deck_Standoff_1", "Pi_Upper_Deck_Standoff_2", "Pi_Upper_Deck_Standoff_3", "Pi_Upper_Deck_Standoff_4", "Separate_5V_BEC_Mounting_Platform", "5V_BEC_Mockup_For_Pi5_And_OAKD_Do_Not_Print", "OAKD_Lite_Front_Camera_Bottom_Shelf", "OAKD_Lite_Front_Camera_Left_Cheek", "OAKD_Lite_Front_Camera_Right_Cheek", "OAKD_Lite_Camera_Rear_Brace", "OAKD_Lite_Clearance_Mockup_Do_Not_Print", "Center_Reference_Marker_Do_Not_Print", "Motor_Pad_1 (1)"
